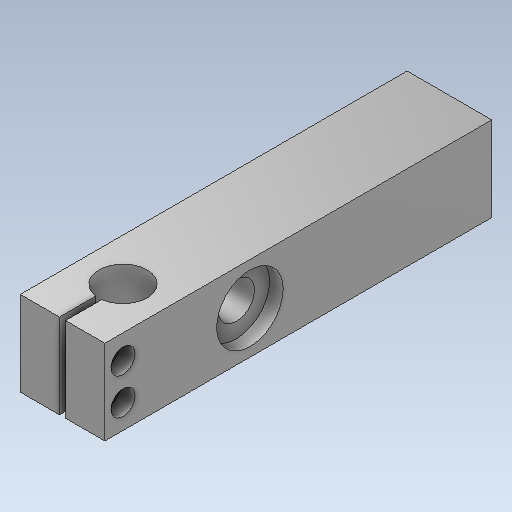
# Autodesk Inventor part: Corner Stand
Saved by Autodesk Inventor 2020 (Build 240168000, 168)
## iProperties
Created: 2020-03-17
Part Number: Corner Stand
Material: Generic
Document SubType Name: Modeling
Designer: DasNick
Density: 1 g/cm^3
Appearance: Default
Author: DasNick
Autodesk Inventor part; units mm, degrees
ref_plane "YZ Plane" through (0, 0, 0) normal (1, 0, 0) x (0, 1, 0)
ref_plane "XZ Plane" through (0, 0, 0) normal (0, 1, 0) x (-1, 0, 0)
ref_plane "XY Plane" through (0, 0, 0) normal (0, 0, 1) x (1, 0, 0)
sketch "Sketch1" plane through (0, 0, 0) normal (0, 0, 1) x (1, 0, 0)
  circle A0 centre (202.1451, 12.6471) radius 3.9688 projected
  circle A1 centre (202.1451, -12.7529) radius 3.9688 projected
  circle A2 centre (176.7451, 12.6471) radius 3.9688 projected
  circle A3 centre (176.7451, -12.7529) radius 3.9688 projected
  line L0 (211.6701, 22.1721) -> (167.2201, 22.1721)
  line L1 (167.2201, 22.1721) -> (167.2201, -22.2779)
  line L2 (167.2201, -22.2779) -> (211.6701, -22.2779)
  line L3 (211.6701, -22.2779) -> (211.6701, 22.1721)
  point P0 (0, 0)
  dimension "d0" = 9.525
  dimension "d1" = 9.525
  dimension "d2" = 44.45
  dimension "d3" = 44.45
  constraints: 8 end point, 2 parallel, 1 horizontal, 1 perpendicular
  measures "d0" distance from line of L3 A0.centre
  measures "d1" distance from line of L0 A0.centre
  measures "d2" distance of L2.end L0.start
  measures "d3" distance of L0.start L0.end
extrude "Extrusion1" add sketch "Sketch1" along normal blind 38.1
sketch "Sketch2" plane through (0, 0, 38.1) normal (0, 0, 1) x (1, 0, 0)
  line L0 (211.6701, -22.2779) -> (211.6701, 22.1721) projected
  line L1 (167.2201, 22.1721) -> (167.2201, -22.2779) projected
  line L2 (211.6701, 22.1721) -> (167.2201, 22.1721)
  line L3 (167.2201, 22.1721) -> (167.2201, -22.2779)
  line L4 (167.2201, -22.2779) -> (211.6701, -22.2779)
  line L5 (211.6701, -22.2779) -> (211.6701, 22.1721)
  point P0 (0, 0)
  constraints: 8 end point, 2 parallel, 1 horizontal, 1 perpendicular
extrude "Extrusion2" add sketch "Sketch2" along normal blind 165.1
sketch "Sketch3" plane through (167.2201, -22.2779, 0) normal (-1, 0, 0) x (0, 0, 1)
  point P0 (0, 22.2779)
sketch "Sketch4" plane through (211.6701, -22.2779, 0) normal (1, 0, 0) x (0, 0, -1)
  circle A0 centre (-127, 22.2779) radius 17.4625
  point P0 (0, 22.2779)
  dimension "d8" = 34.925
  dimension "d11" = 127
  constraints: 1 centre point
  measures "d8" diameter of A0
  measures "d11" distance of point (0, 22.278) A0.centre
extrude "Extrusion3" cut sketch "Sketch4" against normal blind 7.1437
sketch "Sketch5" plane through (204.5263, 0, 127) normal (1, 0, 0) x (0, 0, -1)
  circle A0 centre (0, 0) radius 9.525
  point P0 (127, 0)
  dimension "d12" = 19.05
  constraints: 1 centre point
  measures "d12" diameter of A0
extrude "Extrusion4" cut sketch "Sketch5" against normal blind 50.8
sketch "Sketch6" plane through (167.2201, -22.2779, 0) normal (0, -1, 0) x (1, 0, 0)
  circle A0 centre (22.225, 171.45) radius 12.7
  line L0 (0, 203.2) -> (44.45, 203.2) projected
  point P0 (-167.2201, 0)
  dimension "d15" = 25.4
  dimension "d16" = 31.75
  constraints: 1 centre point
  measures "d15" diameter of A0
  measures "d16" distance from line of L0 A0.centre
extrude "Extrusion5" cut sketch "Sketch6" against normal blind 50.8
sketch "Sketch7" plane through (167.2201, -22.2779, 0) normal (0, -1, 0) x (1, 0, 0)
  line L0 (44.45, 203.2) -> (0, 203.2) projected
  line L1 (23.8125, 203.2) -> (20.6375, 203.2)
  line L2 (20.6375, 203.2) -> (20.6375, 177.8)
  line L3 (20.6375, 177.8) -> (23.8125, 177.8)
  line L4 (23.8125, 177.8) -> (23.8125, 203.2)
  line L5 (44.45, 0) -> (44.45, 203.2) projected
  point P0 (-167.2201, 0)
  dimension "d19" = 3.175
  dimension "d20" = 20.6375
  dimension "d21" = 25.4
  constraints: 8 end point, 2 parallel, 1 horizontal, 1 perpendicular, 1 point on line
  measures "d19" distance of L2.end L3.end
  measures "d20" distance between parallel lines of L5 L4
  measures "d21" distance of L3.end L1.start
extrude "Extrusion6" cut sketch "Sketch7" against normal blind 50.8
sketch "Sketch8" plane through (211.6701, -22.2779, 0) normal (1, 0, 0) x (0, 0, -1)
  circle A0 centre (-193.675, 31.75) radius 6.35
  line L0 (-203.2, 0) -> (-203.2, 44.45) projected
  circle A1 centre (-193.675, 12.7) radius 6.35
  line L1 (0, 44.45) -> (-203.2, 44.45) projected
  line L2 (0, 0) -> (-203.2, 0) projected
  point P0 (0, 22.2779)
  dimension "d24" = 12.7
  dimension "d25" = 9.525
  dimension "d26" = 12.7
  dimension "d27" = 12.7
  dimension "d28" = 12.7
  constraints: 2 centre point
  measures "d24" diameter of A0
  measures "d25" distance from line of L0 A0.centre
  measures "d26" diameter of A1
  measures "d27" distance from line of L1 A0.centre
  measures "d28" distance from line of L2 A1.centre
extrude "Extrusion7" cut sketch "Sketch8" against normal blind 7.9375
sketch "Sketch9" plane through (203.7326, 9.4721, 193.675) normal (1, 0, 0) x (0, 0, -1)
  circle A0 centre (0, 0) radius 6.35 projected
  circle A1 centre (0, 0) radius 3.9688
  circle A2 centre (0, -19.05) radius 6.35 projected
  circle A3 centre (0, -19.05) radius 3.9688
  point P0 (193.675, -9.4721)
  dimension "d31" = 7.9375
  dimension "d32" = 7.9375
  constraints: 2 centre point, 2 coincident
  measures "d31" diameter of A1
  measures "d32" diameter of A3
extrude "Extrusion8" cut sketch "Sketch9" against normal blind 38.1 contours A1 | A3
body "Solid1"
